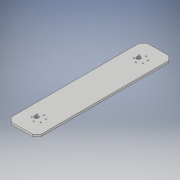
# Autodesk Inventor part: testPart_chassis
Saved by Autodesk Inventor 2019 (Build 230136000, 136)
## iProperties
Created: 2019-09-17
Part Number: testPart_chassis
Material: Generic
Document SubType Name: Modeling
Designer: shrey
Density: 1 g/cm^3
Appearance: Default
Author: shrey
Autodesk Inventor part; units mm, degrees
ref_plane "YZ Plane" through (0, 0, 0) normal (1, 0, 0) x (0, 1, 0)
ref_plane "XZ Plane" through (0, 0, 0) normal (0, 1, 0) x (-1, 0, 0)
ref_plane "XY Plane" through (0, 0, 0) normal (0, 0, 1) x (1, 0, 0)
sketch "Sketch1" plane through (0, 0, 0) normal (0, 1, 0) x (-1, 0, 0)
  line L0 (-44.45, -203.2) -> (44.45, -203.2)
  line L1 (44.45, -203.2) -> (44.45, 203.2)
  line L2 (44.45, 203.2) -> (-44.45, 203.2)
  line L3 (-44.45, 203.2) -> (-44.45, -203.2)
  line L4 (-44.45, -203.2) -> (44.45, 203.2) construction
  line L5 (44.45, -203.2) -> (-44.45, 203.2) construction
  line L6 (0, 203.2) -> (0, -203.2) construction
  circle A0 centre (0, 152.4) radius 15.494 construction
  circle A1 centre (0, 136.906) radius 1.5
  circle A2 centre (13.4182, 144.653) radius 1.5
  circle A3 centre (13.4182, 160.147) radius 1.5
  circle A4 centre (0, 167.894) radius 1.5
  circle A5 centre (-13.4182, 160.147) radius 1.5
  circle A6 centre (-13.4182, 144.653) radius 1.5
  line L7 (0, 0) -> (44.45, 0) construction
  line L8 (0, -203.2) -> (0, 203.2) construction
  circle A7 centre (0, -152.4) radius 15.494 construction
  circle A8 centre (13.4182, -144.653) radius 1.5
  circle A9 centre (13.4182, -160.147) radius 1.5
  circle A10 centre (0, -167.894) radius 1.5
  circle A11 centre (-13.4182, -160.147) radius 1.5
  circle A12 centre (-13.4182, -144.653) radius 1.5
  circle A13 centre (0, -136.906) radius 1.5
  line L9 (0, 152.4) -> (7.112, 152.4) construction
  circle A14 centre (7.112, 152.4) radius 6
  line L10 (0, -152.4) -> (7.112, -152.4) construction
  circle A15 centre (7.112, -152.4) radius 6
  dimension "d3" = 30.988
  dimension "d0" = 406.4
  dimension "d1" = 88.9
  dimension "d2" = 152.4
  dimension "d4" = 3
  dimension "d7" = 360
  dimension "d9" = 7.112
  dimension "d10" = 12
  constraints: 22 end point, 14 centre point, 13 symmetric about line, 5 coincident, 5 midpoint, 4 point on line, 3 horizontal, 2 parallel, 2 vertical alignment, 1 equal radius, 1 perpendicular, 23 other
  measures "d0" distance of L0.end L1.end
  measures "d1" distance of L1.end L2.end
  measures "d2" distance of L7.start point (0, 152.4)
  measures "d4" diameter of A1
  measures "d9" distance of L9.start L9.end
  measures "d10" diameter of A14
extrude "Extrusion1" add sketch "Sketch1" along normal blind 6.35
chamfer "Chamfer1" distance 12.7 angle 45 4 edges at (44.45, 3.175, 203.2) (44.45, 3.175, -203.2) (-44.45, 3.175, 203.2) (-44.45, 3.175, -203.2)
body "Solid1"
